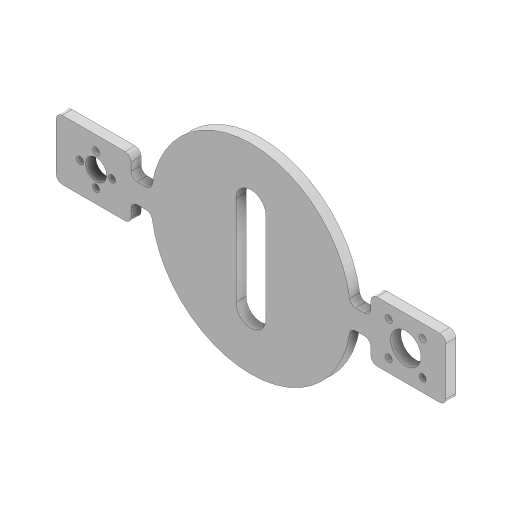
# Autodesk Inventor part: TAPA OPCION 3
Saved by Autodesk Inventor 2024 (Build 280153000, 153)
## iProperties
Created: 2024-05-26
Part Number: TAPA OPCION 3
Material: Generic
Document SubType Name: Modeling
Designer: Jhuliams
Density: 1 g/cm^3
Appearance: Default
Author: Jhuliams
Autodesk Inventor part; units mm, degrees
ref_plane "YZ Plane" through (0, 0, 0) normal (1, 0, 0) x (0, 1, 0)
ref_plane "XZ Plane" through (0, 0, 0) normal (0, 1, 0) x (-1, 0, 0)
ref_plane "XY Plane" through (0, 0, 0) normal (0, 0, 1) x (1, 0, 0)
sketch "Sketch1" plane through (0, 0, 0) normal (0, 0, 1) x (1, 0, 0)
  circle A0 centre (0, 0) radius 50
  line L0 (0, 0) -> (0, 20) construction
  line L1 (2.5, 15) -> (97.5, 15)
  line L2 (97.5, 15) -> (97.5, -15)
  line L3 (97.5, -15) -> (2.5, -15)
  line L4 (2.5, -15) -> (2.5, 15)
  line L5 (2.5, 15) -> (97.5, -15) construction
  line L6 (97.5, 15) -> (2.5, -15) construction
  line L7 (40, 5) -> (60, 5)
  line L8 (60, 5) -> (60, -5)
  line L9 (60, -5) -> (40, -5)
  line L10 (40, -5) -> (40, 5)
  line L11 (40, 5) -> (60, -5) construction
  line L12 (60, 5) -> (40, -5) construction
  line L13 (60, 5) -> (60, 15)
  line L14 (60, -5) -> (60, -15)
  line L15 (-2.5, 15) -> (-97.5, 15)
  line L16 (-97.5, 15) -> (-97.5, -15)
  line L17 (-97.5, -15) -> (-2.5, -15)
  line L18 (-2.5, -15) -> (-2.5, 15)
  line L19 (-2.5, 15) -> (-97.5, -15) construction
  line L20 (-97.5, 15) -> (-2.5, -15) construction
  line L21 (-40, 5) -> (-60, 5)
  line L22 (-60, 5) -> (-60, -5)
  line L23 (-60, -5) -> (-40, -5)
  line L24 (-40, -5) -> (-40, 5)
  line L25 (-40, 5) -> (-60, -5) construction
  line L26 (-60, 5) -> (-40, -5) construction
  line L27 (-60, 5) -> (-60, 15)
  line L28 (-60, -5) -> (-60, -15)
  point P0 (50, 0)
  point P1 (50, 0)
  point P2 (-50, 0)
  point P3 (-50, 0)
  point P4 (49.7494, 5)
  point P5 (49.7494, -5)
  point P6 (-49.7494, -5)
  point P7 (-49.7494, 5)
  dimension "d0" = 100
  dimension "d3" = 20
  dimension "d17" = 95
  dimension "d18" = 30
  dimension "d19" = 20
  dimension "d20" = 10
  constraints: 58 end point, 12 symmetric about line, 5 midpoint, 4 parallel, 4 perpendicular, 4 point on line, 2 horizontal, 1 coincident, 1 vertical, 3 other
  measures "d3" distance of L0.start L0.end
  measures "d17" distance of L2.end L3.end
  measures "d18" distance of L1.end L2.end
  measures "d19" distance of L8.end L9.end
  measures "d20" distance of L7.end L8.end
extrude "Extrusion1" add sketch "Sketch1" along normal blind 5 contours A0 L9 L10 L7 | A0 L7 L8 L9 | L7 L10 L9 A0 L3 L4 L1 | L1 L4 L3 A0 L17 L18 L15 | L13 L1 L2 L3 L14 L8 | L15 L18 L17 A0 L23 L24 L21 | L21 L24 L23 A0 | A0 L23 L22 L21 | L27 L22 L28 L17 L16 L15
sketch "Sketch2" plane through (0, 0, 5) normal (0, 0, 1) x (1, 0, 0)
  line L0 (0, 0) -> (-77.5, 0) construction
  circle A0 centre (-77.5, 0) radius 5.25
  line L1 (0, 0) -> (0, 20) construction
  circle A1 centre (-77.5, 0) radius 8
  circle A2 centre (-69.5, 0) radius 1.75
  circle A3 centre (-77.5, 8) radius 1.75
  circle A4 centre (-85.5, 0) radius 1.75
  circle A5 centre (-77.5, -8) radius 1.75
  circle A6 centre (77.5, 0) radius 12
  line L2 (65, 12.5) -> (90, 12.5)
  line L3 (90, 12.5) -> (90, -12.5)
  line L4 (90, -12.5) -> (65, -12.5)
  line L5 (65, -12.5) -> (65, 12.5)
  line L6 (65, 12.5) -> (90, -12.5) construction
  line L7 (90, 12.5) -> (65, -12.5) construction
  line L8 (90, 12.5) -> (65, -12.5)
  circle A7 centre (85.9853, 8.4853) radius 1.75
  circle A8 centre (69.0147, 8.4853) radius 1.75
  circle A9 centre (69.0147, -8.4853) radius 1.75
  circle A10 centre (85.9853, -8.4853) radius 1.75
  circle A11 centre (77.5, 0) radius 7.6
  dimension "d26" = 16
  dimension "d70" = 24
  dimension "d6" = 77.5
  dimension "d7" = 10.5
  dimension "d8" = 20
  dimension "d27" = 3.5
  dimension "d30" = 360
  dimension "d71" = 25
  dimension "d72" = 25
  dimension "d73" = 3.5
  dimension "d76" = 360
  dimension "d78" = 15.2
  constraints: 18 end point, 10 centre point, 5 coincident, 3 point on line, 2 horizontal, 2 midpoint, 2 parallel, 1 horizontal alignment, 1 perpendicular, 1 symmetric about line, 1 vertical, 23 other
  measures "d6" distance of L0.start L0.end
  measures "d7" diameter of A0
  measures "d8" distance of L0.start L1.end
  measures "d27" diameter of A2
  measures "d71" distance of L3.end L4.end
  measures "d72" distance of L2.end L3.end
  measures "d73" diameter of A7
  measures "d78" diameter of A11
extrude "Extrusion2" cut sketch "Sketch2" against normal blind 7 contours A0 | A1 A2 | A1 A2 | A3 A1 | A1 A3 | A5 A1 | A1 A5 | A4 A1 | A1 A4 | A7 L8 A6 | A6 L8 A7 | A10 A6 | A6 A10 | L8 A7 A6 | A6 A7 L8 | A11 L8 | L8 A11 | A9 L8 A6 | A6 L8 A9 | A8 A6 | A6 A8 | L8 A9 A6 | A6 A9 L8
fillet "Fillet1" radius 3 16 edges at (-60, 5, 2.5) (-60, 15, 2.5) (-49.7494, 5, 2.5) (-60, -5, 2.5) (-60, -15, 2.5) (-49.7494, -5, 2.5) (-97.5, -15, 2.5) (-97.5, 15, 2.5) (97.5, 15, 2.5) (97.5, -15, 2.5) (60, -15, 2.5) (60, 15, 2.5) (60, -5, 2.5) (60, 5, 2.5) (49.7494, 5, 2.5) (49.7494, -5, 2.5)
sketch "Sketch4" plane through (0, 0, 5) normal (0, 0, 1) x (1, 0, 0)
  line L0 (-7.5, 22.5) -> (7.5, 22.5)
  line L1 (7.5, 22.5) -> (7.5, -22.5)
  line L2 (7.5, -22.5) -> (-7.5, -22.5)
  line L3 (-7.5, -22.5) -> (-7.5, 22.5)
  line L4 (-7.5, 22.5) -> (7.5, -22.5) construction
  line L5 (7.5, 22.5) -> (-7.5, -22.5) construction
  circle A0 centre (0, -22.5) radius 7.5
  circle A1 centre (0, 22.5) radius 7.5
  point P0 (0, 0)
  point P1 (7.5, 22.5)
  dimension "d79" = 15
  dimension "d80" = 45
  dimension "d81" = 15
  dimension "d82" = 15
  constraints: 12 end point, 4 midpoint, 2 centre point, 2 parallel, 1 horizontal, 1 perpendicular
  measures "d79" distance of L1.end L2.end
  measures "d80" distance of L0.end L1.end
  measures "d81" diameter of A0
  measures "d82" diameter of A1
extrude "Extrusion3" cut sketch "Sketch4" against normal blind 10
body "Solid1"
